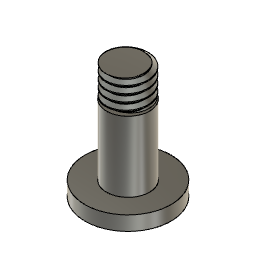
axle yoke (Autodesk Fusion 360 design; units mm, degrees)
Autodesk Fusion 360 part; units mm, degrees
mesh "Mesh1" [no effect] in component "axle yoke"
sketch "axle yoke" plane through (0, 0, 0) normal (0, 0, 1) x (1, 0, 0) in component "axle yoke"
  circle A0 centre (-27.5231, 5.9534) radius 6.0009
  circle A1 centre (-27.5231, 5.9534) radius 3.0025
  constraint concentric A0 A1
extrude "Extrude1" add sketch "axle yoke" along normal blind 2 contours A0 | A1 makes body 1 in component "axle yoke"
extrude "Extrude2" add sketch "axle yoke" along normal blind 11.8 contours A1 bodies 1 in component "axle yoke"
extrude "Extrude3" add 1 faces at (-28.8451, 6.6782, 11.8) along direction (0, 0, 1) blind 4.4 separate body on bodies 1 makes body 2 in component "axle yoke"
thread "Thread1" "ISO Metric profile 6.0 M6x1 6g" major diameter 5.884 minor diameter 4.7435 pitch 1 angle 60 modelled right hand crest width 0.1444 on face at (-24.5243, 5.8037, 14.7333) crest through (-24.5811, 5.9534, 11.55) on bodies 2 in component "axle yoke"
combine "Combine1" operation add target body 2 tool bodies 1 in component "axle yoke"
component "axle yoke" placed x (1, 0, 0) y (0, 1, 0) z (0, 0, 1) at (0, 0, 0)
named bodies: "axle yoke"
